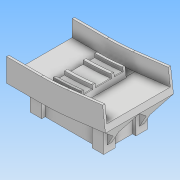
# Autodesk Inventor part: Slope_LowEnd
Saved by Autodesk Inventor 2021 (Build 250183000, 183)
## iProperties
Created: 2021-03-11
Part Number: Slope_LowEnd
Material: 一般
Document SubType Name: Modeling
Designer: kumagai
Density: 1 g/cm^3
Appearance: 既定
Author: kumagai
Autodesk Inventor part; units mm, degrees
ref_plane "YZ Plane" through (0, 0, 0) normal (1, 0, 0) x (0, 1, 0)
derived "SlopeProfile.ipt"
sketch "スケッチ1" plane through (0, 0, 0) normal (0, 0, 1) x (1, 0, 0)
  line L0 (0, 14) -> (0, -14)
  line L1 (-14, 0) -> (14, 0)
  line L2 (-268.75, 0) -> (268.75, 0)
  line L3 (-268.75, 0) -> (268.75, 66)
  line L4 (268.75, 66) -> (268.75, 0)
  line L5 (-31.5879, 61.457) -> (-25.6465, 13.0705)
  line L6 (-134.375, 50.6657) -> (-134.375, 8.5939)
  line L7 (23.2129, 72.7486) -> (28.7067, 28.0077)
  line L8 (-244.2356, 29.1492) -> (-240.1953, -3.7549)
  line L9 (134.375, 89.7324) -> (134.375, 45.3233)
  line L10 (239.1121, 78.5758) -> (241.9591, 55.3901)
  line L11 (-27.6764, 5.7379) -> (-27.6764, -11.9933)
  line L12 (27.6764, 6.5088) -> (27.6764, -13.0212)
  line L13 (-268.75, 0) -> (-295.625, 0)
  line L14 (268.75, 66) -> (295.625, 66)
  line L15 (241.0736, 6.6999) -> (241.0736, -9.2827)
  line L16 (-241.0736, -7.7427) -> (-241.0736, -14.414)
  arc A0 (-280.625, 0) -> (-256.9635, 1.4473) centre (-280.625, 194.1449) ccw
  line L17 (-256.3082, 4.3915) -> (-255.7778, 0.0713)
  line L18 (-280.625, 8.6126) -> (-280.625, -11.6883)
  line L19 (-295.625, 14.7784) -> (-295.625, -11.568)
  line L20 (255.3892, 69.0933) -> (256.9398, 56.465)
  line L21 (280.625, 71.1514) -> (280.625, 58.4982)
  line L22 (295.625, 71.9522) -> (295.625, 60.0478)
  arc A1 (280.625, 66) -> (256.9635, 64.5527) centre (280.625, -128.1449) ccw
  line L23 (-13.2739, 35.3851) -> (-12.039, 25.3288)
  line L24 (-43.1495, 32.5373) -> (-41.4451, 18.6566)
  line L25 (12.2235, 39.1691) -> (13.7539, 26.7059)
  line L26 (41.8424, 44.108) -> (43.6336, 29.5201)
  point P0 (0, 0)
  point P1 (-241.0736, 3.3984)
  point P2 (-27.6764, 29.6016)
  point P3 (27.6764, 36.3984)
  point P4 (241.0736, 62.6016)
  point P5 (134.375, 49.5)
  point P6 (-134.375, 16.5)
ref_plane "作業平面1" through (-241.0736, 3.3984, 0) normal (0.9925454, 0.1218753, 0) x (-0.1218753, 0.9925454, 0)
sketch "スケッチ2" plane through (-241.0736, 3.3984, 0) normal (0.9925454, 0.1218753, 0) x (-0.1218753, 0.9925454, 0)
  line L0 (-5.2, 19) -> (-5.2, -19)
  line L1 (-5.2, -19) -> (3.2, -19)
  line L2 (3.2, -19) -> (3.2, -17)
  line L3 (3.2, -17) -> (0, -17)
  line L4 (0, -17) -> (0, -9.3)
  line L5 (0, -9.3) -> (3.2, -9.3)
  line L6 (3.2, -9.3) -> (3.2, -6.9)
  line L7 (3.2, -6.9) -> (0, -6.9)
  line L8 (0, -6.9) -> (0, 6.9)
  line L9 (0, 6.9) -> (3.2, 6.9)
  line L10 (3.2, 6.9) -> (3.2, 9.3)
  line L11 (3.2, 9.3) -> (0, 9.3)
  line L12 (0, 9.3) -> (0, 17)
  line L13 (0, 17) -> (3.2, 17)
  line L14 (3.2, 17) -> (3.2, 19)
  line L15 (3.2, 19) -> (-5.2, 19)
  line L16 (25.9442, 0) -> (-7.2071, 0) projected
  line L17 (-5.2, 27.5) -> (-5.2, -27.5)
  line L18 (-5.2, -27.5) -> (9, -27.5)
  line L19 (9, -27.5) -> (9, -29.5)
  line L20 (9, -29.5) -> (-11, -29.5)
  line L21 (-11, -29.5) -> (-11, 29.5)
  line L22 (-11, 29.5) -> (9, 29.5)
  line L23 (9, 29.5) -> (9, 27.5)
  line L24 (9, 27.5) -> (-5.2, 27.5)
  line L25 (-11, 29.5) -> (-22.3278, 16)
  line L26 (-22.3278, 16) -> (-31, 16)
  line L27 (-31, 16) -> (-31, 12)
  line L28 (-31, 12) -> (-21.0692, 12)
  line L29 (-21.0692, 12) -> (-11, 0)
  line L30 (-11, 0) -> (-21.0692, -12)
  line L31 (-21.0692, -12) -> (-31, -12)
  line L32 (-31, -12) -> (-31, -16)
  line L33 (-31, -16) -> (-22.3278, -16)
  line L34 (-22.3278, -16) -> (-11, -29.5)
  point P0 (-32.754, 0)
  point P1 (0, 0)
  point P2 (-5.2, -19)
  point P3 (-5.2, 19)
  dimension "d25" = 38
  dimension "d26" = 18.6
  dimension "d27" = 2
  dimension "d28" = 2.4
  dimension "d29" = 3.2
  dimension "d30" = 8.4
  dimension "d46" = 59
  dimension "d47" = 2
  dimension "d48" = 20
  dimension "d49" = 5.8
  dimension "d50" = 5.8
  dimension "d51" = 40
  dimension "d52" = 40
  dimension "d53" = 4
  dimension "d54" = 32
  dimension "d55" = 20
  constraints: 68 end point, 15 point on line, 10 perpendicular, 4 horizontal, 4 vertical, 2 midpoint, 1 collinear, 10 other
  measures "d25" distance between parallel lines of L1 L15
  measures "d26" distance between parallel lines of L5 L11
  measures "d27" distance between parallel lines of L15 L13
  measures "d28" distance between parallel lines of L9 L11
  measures "d29" distance between parallel lines of L12 L14
  measures "d30" distance between parallel lines of L0 L14
  measures "d46" distance between parallel lines of L20 L22
  measures "d47" distance between parallel lines of L22 L24
  measures "d48" distance between parallel lines of L21 L23
  measures "d49" distance between parallel lines of L23 L14
  measures "d50" distance between parallel lines of L21 L17
  measures "d51" angle of L25 L21
  measures "d52" angle of L21 L29
  measures "d53" distance between parallel lines of L28 L26
  measures "d54" distance between parallel lines of L33 L26
  measures "d55" distance between parallel lines of L32 L21
sketch "スケッチ3" plane through (0, 0, 0) normal (0, 0, 1) x (1, 0, 0)
  line L0 (-268.75, 0) -> (268.75, 66) projected
  line L1 (-241.4636, 6.5745) -> (-240.4399, -1.7628) projected
  line L2 (-256.3082, 4.3915) -> (-255.7778, 0.0713) projected
  arc A0 (-280.625, 0) -> (-256.9635, 1.4473) centre (-280.625, 194.1449) ccw projected
  line L3 (-256.9635, 1.4473) -> (-226.1855, 5.2265)
  line L4 (-280.625, 0) -> (-310.625, 0)
  point P0 (0, 0)
  point P1 (-295.625, 0)
  dimension "PrinterOffset" = 0
  dimension "d33" = 15
  dimension "d58" = 15
  constraints: 4 end point, 1 midpoint, 1 point on line, 1 tangent
  measures "d33" distance from line of L3.end L1
  measures "d58" distance of L4.end point (-295.625, 0)
sweep "スイープ1" add profiles "スケッチ2" path "スケッチ3" path curves L3 A0 L4
extrude "押し出し1" cut sketch "スケッチ2" along normal blind 20 and the other way blind 15 contours L15 L14 L13 L12 L11 L10 L9 L8 L16 L0 | L16 L8 L7 L6 L5 L4 L3 L2 L1 L0
sketch "スケッチ5" plane through (-310.625, -11, -29.5) normal (-1, 0, 0) x (0, 0, 1)
  line L0 (10.5, 14.2) -> (10.5, 5.8) projected
  line L1 (48.5, 5.8) -> (48.5, 14.2) projected
  line L2 (10.5, 5.8) -> (48.5, 5.8)
  line L3 (48.5, 5.8) -> (48.5, 14.2)
  line L4 (48.5, 14.2) -> (10.5, 14.2)
  line L5 (10.5, 14.2) -> (10.5, 5.8)
  point P0 (29.5, 11)
  dimension "PrinterOffset" = 0
  constraints: 8 end point
extrude "押し出し3" cut sketch "スケッチ5" against normal blind 30
ref_plane "作業平面2" through (0, -33, 0) normal (0, 1, 0) x (-1, 0, 0)
sketch "スケッチ6" plane through (0, -33, 0) normal (0, 1, 0) x (-1, 0, 0)
  line L0 (-416.875, 0) -> (431.875, 0) projected
  line L1 (290.625, -19) -> (300.625, -19)
  line L2 (300.625, -19) -> (300.625, -9)
  line L3 (300.625, -9) -> (290.625, -9)
  line L4 (290.625, -9) -> (290.625, -19)
  line L5 (236.875, -19) -> (246.875, -19)
  line L6 (246.875, -19) -> (246.875, -9)
  line L7 (246.875, -9) -> (236.875, -9)
  line L8 (236.875, -9) -> (236.875, -19)
  line L9 (290.625, 19) -> (300.625, 19)
  line L10 (300.625, 19) -> (300.625, 9)
  line L11 (300.625, 9) -> (290.625, 9)
  line L12 (290.625, 9) -> (290.625, 19)
  line L13 (236.875, 19) -> (246.875, 19)
  line L14 (246.875, 19) -> (246.875, 9)
  line L15 (246.875, 9) -> (236.875, 9)
  line L16 (236.875, 9) -> (236.875, 19)
  line L17 (246.875, -16) -> (290.625, -16)
  line L18 (290.625, -16) -> (290.625, -12)
  line L19 (290.625, -12) -> (246.875, -12)
  line L20 (246.875, -12) -> (246.875, -16)
  line L21 (246.875, 12) -> (290.625, 12)
  line L22 (290.625, 12) -> (290.625, 16)
  line L23 (290.625, 16) -> (246.875, 16)
  line L24 (246.875, 16) -> (246.875, 12)
  line L25 (243.875, 9) -> (239.875, 9)
  line L26 (239.875, 9) -> (239.875, -9)
  line L27 (239.875, -9) -> (243.875, -9)
  line L28 (243.875, -9) -> (243.875, 9)
  line L29 (293.625, -9) -> (297.625, -9)
  line L30 (297.625, -9) -> (297.625, 9)
  line L31 (297.625, 9) -> (293.625, 9)
  line L32 (293.625, 9) -> (293.625, -9)
  point P0 (0, 0)
  point P1 (295.625, 0)
  point P2 (295.625, 0)
  point P3 (295.625, 0)
  dimension "PrinterOffset" = 0
  dimension "d63" = 10
  dimension "d64" = 10
  dimension "d65" = 53.75
  dimension "d66" = 38
  dimension "d68" = 10
  dimension "d69" = 3
  dimension "d71" = 3
  dimension "d72" = 3
  dimension "d73" = 3
  dimension "d74" = 3
  dimension "d75" = 3
  dimension "d76" = 5
  constraints: 64 end point, 9 collinear, 8 symmetric about line, 6 point on line, 1 horizontal, 1 vertical, 2 other
  measures "d63" distance between parallel lines of L2 L4
  measures "d64" distance between parallel lines of L8 L6
  measures "d65" distance between parallel lines of L2 L6
  measures "d66" distance between parallel lines of L9 L1
  measures "d68" distance between parallel lines of L1 L3
  measures "d69" distance between parallel lines of L5 L17
  measures "d71" distance between parallel lines of L7 L19
  measures "d72" distance between parallel lines of L6 L28
  measures "d73" distance between parallel lines of L8 L26
  measures "d74" distance between parallel lines of L4 L32
  measures "d75" distance between parallel lines of L2 L30
  measures "d76" distance from line of point (295.625, 0) L18
extrude "押し出し4" add sketch "スケッチ6" along normal up to next contours L26 L15 L28 L0 | L0 L28 L7 L26 | L15 L16 L13 L14 | L7 L6 L5 L8 | L32 L11 L30 L0 | L0 L30 L3 L32 | L11 L12 L9 L10 | L3 L2 L1 L4 | L19 L4 L17 L6 | L14 L23 L12 L21
sketch "スケッチ7" plane through (0, 0, 0) normal (0, 0, 1) x (1, 0, 0)
  line L0 (-300.625, -31) -> (-310.625, -11)
  line L1 (-310.625, -11) -> (-310.625, -31)
  line L2 (-310.625, -31) -> (-300.625, -31)
  line L3 (-224.8448, -5.6915) -> (-219.8448, -5.6915)
  line L4 (-219.8448, -5.6915) -> (-219.8448, -27.3189)
  line L5 (-219.8448, -27.3189) -> (-236.875, -27.3189)
  line L6 (-236.875, -27.3189) -> (-224.8448, -5.6915)
  point P0 (0, 0)
  dimension "d79" = 5
  constraints: 14 end point, 3 horizontal, 2 vertical
  measures "d79" distance of L3.start L3.end
extrude "押し出し5" cut sketch "スケッチ7" along normal through all both and the other way through all
equation "\"d25\" = RailWidth"
equation "\"d26\" = InsideWidth"
equation "\"d27\" = OuterWall"
equation "\"d28\" = InnerWall"
equation "\"d29\" = RailDepth"
equation "\"d30\" = RailHeight"
equation "\"d49\" = d50"
equation "\"d37\" = ConnectorLength"
equation "\"d65\" = 0.25 * StraightLength"
equation "\"d66\" = RailWidth"
equation "\"d71\" = d69"
equation "\"d72\" = d69"
equation "\"d73\" = d69"
equation "\"d74\" = d69"
equation "\"d75\" = d69"
equation "\"RailWidth\" = 38"
equation "\"InsideWidth\" = 18.6"
equation "\"OuterWall\" = 2"
equation "\"InnerWall\" = 2.4"
equation "\"RailDepth\" = 3.2"
equation "\"RailHeight\" = 8.4"
equation "\"ConnectorLength\" = 15"
equation "\"StraightLength\" = 215"
